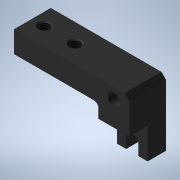
# Autodesk Inventor part: MCHA-20_(g)
Saved by Autodesk Inventor 2021 (Build 250183000, 183)
## iProperties
Created: 2025-07-26
Part Number: MCHA-20_(g)
Material: Generic
Catalog Web Link: www.cadenas.de
Description: MCHA-grip-Grippers
Vendor: MINDMAN
Document SubType Name: Modeling
Designer: psAdmin
Manufacturer: MINDMAN
Mass: 3.89107 g
Surface Area: 23.3352 cm^2
Volume: 3.89107 cm^3
Density: 1 g/cm^3
Appearance: PSOLRGB-175-175-175
Category: PARTsolutions
Company: MINDMAN
Title: MCHA-20_(g)
Author: Cadenas PARTsolutions
Comments: Grippers
PSOL_IDENT_0: {$CADENAS_DATA/23d-libs/mindman/end_of_arm_tooling/grippers/angular_gripper/mcha/mcha_grip.prj},165
PSOL_IDENT_1: {VTYP=3D},{NB=MCHA-20_(g)},{LINA=MCHA-20_(g)},{NN=MCHA-grip},{DATE=08.11.2024 07:05:21},{GEOMDATE=06
PSOL_IDENT_2: .06.2024 03:30:38},{VERSION=},{LINEID=30},{WBVAR=},{WBNUMERIC=}  {NB=MCHA-20_(g)},{LINA=MCHA-20_(g)}
PSOL_IDENT_3: ,{KT=DUMMY},{IDNR=MIN},{MODEL=MCHA},{TUBE=20},{CODE=MCHA-20},{A=22.0},{B=4},{C=10},{D=12},{E=40.1},{
PSOL_IDENT_4: F=18},{G=30},{H=8.0},{I=13.0},{J=25.0},{K=45},{L=25.0},{M=39.5},{N=32.5},{O=16.0},{P=19.0},{Q=50.0},
PSOL_IDENT_5: {R=16},{S=26},{T=35},{UU=M5 x 8depth},{VV=M5 x 8depth},{WW=M5 x 12depth},{XX=M5 x 5depth},{YY=M4},{Z=
PSOL_IDENT_6: 7},{ZZ=3.5},{A1=29.2},{B1=0.0},{C1=0.1},{A2=29.2},{B2=1.9},{C2=0.0}
NB: MCHA-20_(g)
NN: MCHA-grip
NT: Grippers
NBSYN: $CODE._(g)
LINA: MCHA-20_(g)
CATALOG: MINDMAN
IDNR: 0
MODEL: MCHA
TUBE: 20
A: 22
B: 4
C: 10
D: 12
E: 40.1
F: 18
G: 30
H: 8
I: 13
J: 25
K: 45
L: 25
M: 39.5
N: 32.5
O: 16
P: 19
Q: 50
R: 16
S: 26
T: 35
UU: M5 x 8depth
VV: M5 x 8depth
WW: M5 x 12depth
XX: M5 x 5depth
YY: M4
Z: 7
ZZ: 3.5
A1: 29.2
B1: 0
C1: 0.1
A2: 29.2
B2: 1.9
C2: 0
SUPPLIER: MINDMAN
ARTICLENO: MCHA-20_(g)
BOMINFO: MCHA-20_(g)
CREATOR: CADENAS GmbH
Autodesk Inventor part; units mm, degrees
sketch "Sketch_1" plane through (0, 0, 0) normal (0, 0, 1) x (1, 0, 0)
  line L0 (0, 14.5) -> (26, 14.5)
  arc A0 (27.5, 13) -> (26, 14.5) centre (26, 13) ccw
  line L1 (27.5, 13) -> (27.5, 0)
  line L2 (27.5, 0) -> (30.5, 0)
  line L3 (30.5, 0) -> (30.5, 3.5)
  arc A1 (34.5, 3.5) -> (30.5, 3.5) centre (32.5, 3.5) ccw
  line L4 (34.5, 3.5) -> (34.5, 0)
  line L5 (34.5, 0) -> (37.5, 0)
  line L6 (37.5, 0) -> (37.5, 20)
  line L7 (37.5, 20) -> (36, 21.5)
  line L8 (36, 21.5) -> (0, 21.5)
  line L9 (0, 21.5) -> (0, 14.5)
  constraints: 20 end point, 4 point on circle, 2 centre point
extrude "Extrusion1" add sketch "Sketch_1" along normal blind 12
sketch "Sketch2" plane through (0, 0, 0) normal (0, 0, -1) x (-1, 0, 0)
  point P0 (-32.5, 18)
hole "Hole1" at (32.5, 18, 0) direction (0, 0, 1) diameter 4 depth 12
sketch "Sketch_3" plane through (4, 0, 0) normal (1, 0, 0) x (0, 0, -1)
  line L0 (-6, 14.5) -> (-6, 21.5)
  line L1 (-6, 21.5) -> (-4, 21.5)
  line L2 (-4, 21.5) -> (-4.379, 21.121)
  line L3 (-4.379, 21.121) -> (-4.379, 14.879)
  line L4 (-4.379, 14.879) -> (-4, 14.5)
  line L5 (-4, 14.5) -> (-6, 14.5)
  line L6 (-6, 14.5) -> (-6, 21.5)
  constraints: 14 end point
revolve "Revolution1" cut sketch "Sketch_3" angle 360 about axis through (4, 14.5, 6) along (0, -1, 0)
thread "Thread1" size "M4x0.7" class "6H" standard "ISO Metric profile" full length
sketch "Sketch_4" plane through (14, 0, 0) normal (1, 0, 0) x (0, 0, -1)
  line L0 (-6, 14.5) -> (-6, 21.5)
  line L1 (-6, 21.5) -> (-4, 21.5)
  line L2 (-4, 21.5) -> (-4.379, 21.121)
  line L3 (-4.379, 21.121) -> (-4.379, 14.879)
  line L4 (-4.379, 14.879) -> (-4, 14.5)
  line L5 (-4, 14.5) -> (-6, 14.5)
  line L6 (-6, 14.5) -> (-6, 21.5)
  constraints: 14 end point
revolve "Revolution2" cut sketch "Sketch_4" angle 360 about axis through (14, 14.5, 6) along (0, -1, 0)
thread "Thread2" size "M4x0.7" class "6H" standard "ISO Metric profile" full length
sketch "Sketch_6" plane through (0, 0, 6) normal (0, 0, 1) x (1, 0, 0)
  line L0 (27.5, 0) -> (37.5, 0)
  line L1 (37.5, 0) -> (37.5, 10)
  line L2 (37.5, 10) -> (27.5, 10)
  line L3 (27.5, 10) -> (27.5, 0)
  constraints: 8 end point
extrude "Extrusion2" cut sketch "Sketch_6" along normal blind 6
ref_plane "body_XY" through (32.5, 18, 6) normal (0, 0, 1) x (1, 0, 0)
ref_plane "body_YZ" through (32.5, 18, 6) normal (1, 0, 0) x (0, 1, 0)
ref_plane "body_ZX" through (32.5, 18, 6) normal (0, 1, 0) x (0, 0, 1)
body "Solid1"
